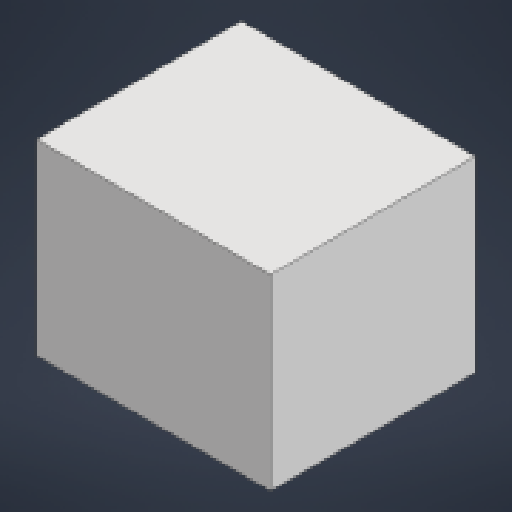
# Autodesk Inventor part: PCB_Housing_04_V3
Saved by Autodesk Inventor 2026.2 (Build 302298000, 298)
## iProperties
Created: 2026-03-10
Part Number: PCB_Housing_04_V3
Material: Generic
Document SubType Name: Modeling
Designer: vckot
Density: 1 g/cm^3
Appearance: Default
Author: vckot
Autodesk Inventor part; units mm, degrees
ref_plane "YZ Plane" through (0, 0, 0) normal (1, 0, 0) x (0, 1, 0)
ref_plane "XZ Plane" through (0, 0, 0) normal (0, 1, 0) x (-1, 0, 0)
ref_plane "XY Plane" through (0, 0, 0) normal (0, 0, 1) x (1, 0, 0)
sketch "Sketch1" plane through (0, 0, 0) normal (0, 1, 0) x (-1, 0, 0)
  line L0 (-10, 8.75) -> (10, 8.75)
  line L1 (10, 8.75) -> (10, -8.75)
  line L2 (10, -8.75) -> (-10, -8.75)
  line L3 (-10, -8.75) -> (-10, 8.75)
  line L4 (-10, 8.75) -> (10, -8.75) construction
  line L5 (10, 8.75) -> (-10, -8.75) construction
  point P0 (0, 0)
  dimension "d0" = 20
  dimension "d1" = 17.5
  constraints: 12 end point, 2 midpoint, 2 parallel, 1 horizontal, 1 perpendicular
  measures "d0" distance of L1.end L2.end
  measures "d1" distance of L0.end L1.end
extrude "Extrusion1" add sketch "Sketch1" along normal mid plane 16
body "Solid1"
